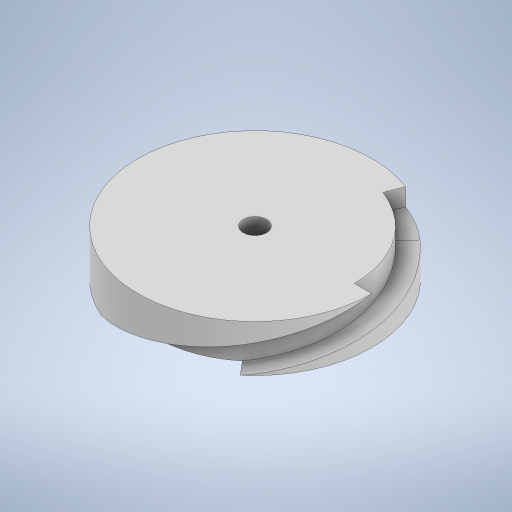
# Autodesk Inventor part: pot dropper
Saved by Autodesk Inventor 2023 (Build 270158000, 158)
## iProperties
Created: 2023-01-12
Part Number: pot dropper
Material: Generic
Document SubType Name: Modeling
Designer: jsmon
Density: 1 g/cm^3
Appearance: Default
Author: jsmon
Autodesk Inventor part; units mm, degrees
ref_plane "XZ Plane" through (0, 0, 0) normal (0, 1, 0) x (-1, 0, 0)
ref_plane "XY Plane" through (0, 0, 0) normal (0, 0, 1) x (1, 0, 0)
sketch "Sketch1" plane through (0, 0, 0) normal (0, 1, 0) x (-1, 0, 0)
  circle A0 centre (0, 0) radius 25.4
  dimension "d0" = 50.8
  constraints: 1 centre point, 1 coincident
  measures "d0" diameter of A0
extrude "Extrusion1" add sketch "Sketch1" along normal blind 10.16
ref_plane "Work Plane1" through (25.4, 0, 0) normal (1, 0, 0) x (0, 1, 0)
sketch "Sketch3" plane through (25.4, 0, 0) normal (1, 0, 0) x (0, 1, 0)
  line L0 (10.16, 0) -> (10.16, 25.4) projected
  line L1 (10.16, 0) -> (0, 50.4021)
  line L2 (10.16, 0) -> (11.8522, -8.3949)
  line L3 (8.3054, -30.7748) -> (11.8522, -8.3949)
  line L4 (6.985, -21.844) -> (6.985, -25.4) projected
  line L5 (0, -25.4) -> (0, 25.4) projected
  line L6 (0, 25.4) -> (0, 50.4021)
  line L7 (8.3054, -30.7748) -> (7.6704, -30.7748)
  line L8 (7.6704, -30.7748) -> (0, 22.2126)
  line L9 (0, 25.4) -> (0, 22.2126)
  point P0 (0, 0)
  dimension "d7" = 0.635
  constraints: 14 end point, 2 collinear, 2 point on line, 1 horizontal
  measures "d7" distance of L3.start L7.end
emboss "Emboss1" sketch "Sketch3" operation cut depth 3.81 direction (1, 0, 0) wrap yes faces at (-25.3176, 6.7733, -2.0439)
sketch "Sketch4" plane through (0, 10.16, 0) normal (0, 1, 0) x (1, 0, 0)
  arc A0 (21.59, 0) -> (15.784, 14.7307) centre (0, 0) ccw projected
  arc A1 (18.5694, 17.3302) -> (25.4, 0) centre (0, 0) ccw projected
  line L0 (9.1112, 23.7096) -> (7.858, 21.467)
  line L1 (7.5892, 20.2122) -> (8.9285, 23.779) projected
  arc A2 (15.784, 14.7307) -> (7.5892, 20.2122) centre (-0.7242, -1.0826) ccw
  arc A3 (18.5694, 17.3302) -> (8.9285, 23.779) centre (0, 0) ccw
  line L2 (15.784, 14.7307) -> (18.5694, 17.3302)
  constraints: 5 point on circle, 4 end point, 2 centre point, 1 concentric
extrude "Extrusion3" cut sketch "Sketch4" against normal blind 3.81
sketch "Sketch5" plane through (0, 10.16, 0) normal (0, 1, 0) x (1, 0, 0)
  circle A0 centre (0, 0) radius 2.54
  dimension "d12" = 5.08
  constraints: 1 centre point, 1 coincident
  measures "d12" diameter of A0
extrude "Extrusion4" cut sketch "Sketch5" against normal blind 45.4025
body "Solid1"
